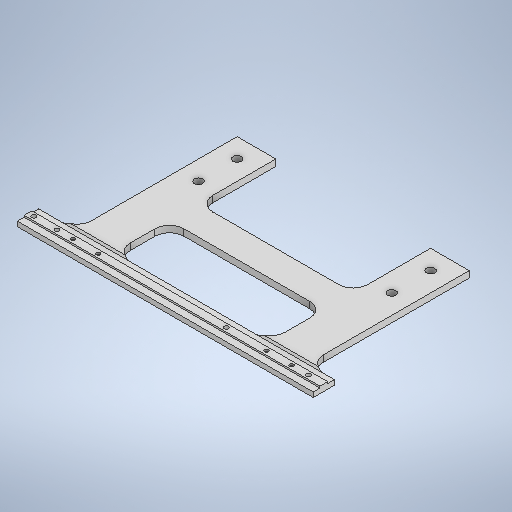
# Autodesk Inventor part: ER_Halterung_Verschraubeinheit
Saved by Autodesk Inventor 2025.2 (Build 292293000, 293)
## iProperties
Created: 2025-06-21
Part Number: ER_Halterung_Verschraubeinheit
Material: Generic
Document SubType Name: Modeling
Designer: Erik
Density: 1 g/cm^3
Appearance: Default
Author: Erik
Autodesk Inventor part; units mm, degrees
ref_plane "YZ Plane" through (0, 0, 0) normal (1, 0, 0) x (0, 1, 0)
ref_plane "XZ Plane" through (0, 0, 0) normal (0, 1, 0) x (-1, 0, 0)
ref_plane "XY Plane" through (0, 0, 0) normal (0, 0, 1) x (1, 0, 0)
sketch "Sketch1" plane through (0, 0, 0) normal (0, 1, 0) x (-1, 0, 0)
  line L0 (-153, 11) -> (153, 11)
  line L1 (153, 11) -> (153, -11)
  line L2 (153, -11) -> (-153, -11)
  line L3 (-153, -11) -> (-153, 11)
  line L4 (-153, 11) -> (153, -11) construction
  line L5 (153, 11) -> (-153, -11) construction
  point P0 (0, 0)
  dimension "d0" = 306
  dimension "d1" = 22
  constraints: 12 end point, 2 midpoint, 2 parallel, 1 horizontal, 1 perpendicular
  measures "d0" distance of L0.start L0.end
  measures "d1" distance of L0.end L1.end
extrude "Extrusion1" add sketch "Sketch1" along normal blind 5
sketch "Sketch2" plane through (0, 5, 0) normal (0, 1, 0) x (1, 0, 0)
  line L0 (-153, 11) -> (-153, -11) projected
  line L1 (153, -4) -> (-153, -4)
  line L2 (-153, -4) -> (-153, 4)
  line L3 (-153, 4) -> (153, 4)
  line L4 (153, 4) -> (153, -4)
  line L5 (153, -4) -> (-153, 4) construction
  line L6 (-153, -4) -> (153, 4) construction
  point P0 (0, 0)
  point P1 (-153, -4)
  dimension "d4" = 8
  constraints: 12 end point, 2 midpoint, 2 parallel, 1 horizontal, 1 perpendicular, 1 point on line
  measures "d4" distance between parallel lines of L3 L1
extrude "Extrusion2" add sketch "Sketch2" along normal blind 1.7
sketch "Sketch3" plane through (0, 0, 0) normal (0, -1, 0) x (1, 0, 0)
  line L0 (153, -11) -> (-153, -11) projected
  line L1 (-113, -11) -> (-73, -11)
  line L2 (-73, -11) -> (-73, -71)
  line L3 (-73, -71) -> (-113, -71)
  line L4 (-113, -71) -> (-113, -11)
  line L5 (-153, -11) -> (-153, 11) projected
  line L6 (0, 27.4) -> (0, -87.4) projected
  line L7 (113, -11) -> (73, -11)
  line L8 (153, -11) -> (153, 11)
  line L9 (113, -11) -> (73, -11)
  line L10 (73, -11) -> (73, -71)
  line L11 (73, -71) -> (113, -71)
  line L12 (113, -71) -> (113, -11)
  point P0 (0, 0)
  point P1 (-73, -11)
  point P2 (153, 0)
  dimension "d7" = 40
  dimension "d8" = 60
  dimension "d9" = 40
  dimension "d23" = 40
  dimension "d24" = 60
  dimension "d25" = 40
  constraints: 20 end point, 4 parallel, 3 symmetric about line, 2 horizontal, 2 perpendicular, 2 point on line, 1 midpoint
  measures "d7" distance of L2.end L3.end
  measures "d8" distance of L1.end L2.end
  measures "d9" distance between parallel lines of L5 L4
  measures "d23" distance of L11.end L10.end
  measures "d24" distance of L10.end L9.end
  measures "d25" distance from line of point (153, 0) L12
extrude "Extrusion3" [suppressed]
sketch "Sketch4" plane through (0, 0, 0) normal (0, -1, 0) x (1, 0, 0)
  line L0 (-153, -11) -> (-153, 11) projected
  point P0 (0, 0)
  point P1 (-147, 0)
  point P2 (-123, 0)
  point P3 (52, 0)
  point P4 (137, 0)
  dimension "d12" = 6
  dimension "d13" = 24
  dimension "d14" = 175
  dimension "d15" = 85
  measures "d12" distance from line of L0 point (-147, 0)
  measures "d13" distance of point (-123, 0) point (-147, 0)
  measures "d14" distance of point (52, 0) point (-123, 0)
  measures "d15" distance of point (137, 0) point (52, 0)
hole "Hole1" at (-147, 0, 0) at (-123, 0, 0) at (52, 0, 0) at (137, 0, 0) direction (0, 1, 0) diameter 4.5 end through all
sketch "Sketch5" plane through (0, 0, 0) normal (0, -1, 0) x (1, 0, 0)
  line L0 (153, 11) -> (153, -11) projected
  line L1 (-153, -11) -> (-153, 11) projected
  point P0 (0, 0)
  point P1 (-80.3, 0)
  point P2 (-106.3, 0)
  point P3 (-153, 0)
  dimension "d27" = 26
  dimension "d38" = 46.7
  constraints: 1 midpoint
  measures "d27" distance of point (-80.3, 0) point (-106.3, 0)
  measures "d38" distance of point (-153, 0) point (-106.3, 0)
hole "Hole2" at (-80.3, 0, 0) at (-106.3, 0, 0) direction (0, 1, 0) diameter 4.134 depth 6.7 thread size "M5x0.8" class "6H" standard "ISO Metric profile"
pattern_linear "Rectangular Pattern1" count 2 spacing 200 along (1, 0, 0) of "Hole2"
sketch "Sketch6" plane through (0, 0, 0) normal (0, -1, 0) x (1, 0, 0)
  line L0 (-113.3, 11) -> (-73.3, 11)
  line L1 (-73.3, 11) -> (-73.3, -176.642)
  line L2 (-73.3, -176.642) -> (-113.3, -176.642)
  line L3 (-113.3, -176.642) -> (-113.3, 11)
  circle A0 centre (-123, 0) radius 2.25 projected
  line L4 (-153, 11) -> (153, 11) projected
  line L5 (86.7, 11) -> (126.7, 11)
  line L6 (126.7, 11) -> (126.7, -176.642)
  line L7 (126.7, -176.642) -> (86.7, -176.642)
  line L8 (86.7, -176.642) -> (86.7, 11)
  circle A1 centre (119.7, 0) radius 2.067 projected
  circle A2 centre (-106.3, 0) radius 2.067 projected
  point P0 (0, 0)
  dimension "d39" = 40
  dimension "d41" = 187.642
  dimension "d42" = 40
  dimension "d44" = 7
  dimension "d47" = 7
  constraints: 16 end point, 4 parallel, 3 collinear, 2 horizontal, 2 perpendicular, 1 point on line
  measures "d39" distance of L1.end L2.end
  measures "d41" distance between parallel lines of L0 L2
  measures "d42" distance of L6.end L7.end
  measures "d44" distance from line of A1.centre L6
  measures "d47" horizontal distance of L0.start A2.centre
extrude "Extrusion4" add sketch "Sketch6" against normal up to surface (5 mm away) contours L0 L1 L2 L3 | L4 L6 L7 L8 | A1 | A2
sketch "Sketch7" plane through (0, 0, 0) normal (0, -1, 0) x (1, 0, 0)
  line L0 (-73.3, -176.642) -> (-73.3, -11) projected
  line L1 (-113.3, -176.642) -> (-73.3, -176.642) projected
  point P0 (0, 0)
  point P1 (-93.3, -156.642)
  point P2 (-93.3, -116.642)
  dimension "d48" = 20
  dimension "d49" = 20
  dimension "d50" = 20
  dimension "d51" = 40
  measures "d48" distance from line of L0 point (-93.3, -156.642)
  measures "d49" distance from line of L0 point (-93.3, -116.642)
  measures "d50" distance from line of L1 point (-93.3, -156.642)
  measures "d51" distance of point (-93.3, -156.642) point (-93.3, -116.642)
hole "Hole3" at (-93.3, 0, -156.642) at (-93.3, 0, -116.642) direction (0, 1, 0) diameter 8.6 end through all
pattern_linear "Rectangular Pattern2" count 2 spacing 200 along (1, 0, 0) of "Hole3"
sketch "Skizze8" plane through (0, 5, 0) normal (0, 1, 0) x (1, 0, 0)
  circle A0 centre (106.7, 116.642) radius 4.3 projected
  circle A1 centre (106.7, 156.642) radius 4.3 projected
  circle A2 centre (-93.3, 116.642) radius 4.3 projected
  circle A3 centre (-93.3, 156.642) radius 4.3 projected
  line L0 (-153, 4) -> (153, 4) projected
  line L1 (153, 4) -> (153, 11) projected
  line L2 (153, 11) -> (126.7, 11) projected
  line L3 (126.7, 176.642) -> (126.7, 11) projected
  line L4 (86.7, 176.642) -> (126.7, 176.642) projected
  line L5 (86.7, 11) -> (86.7, 176.642) projected
  line L6 (86.7, 11) -> (-73.3, 11) projected
  line L7 (-73.3, 176.642) -> (-73.3, 11) projected
  line L8 (-113.3, 176.642) -> (-73.3, 176.642) projected
  line L9 (-113.3, 11) -> (-113.3, 176.642) projected
  line L10 (-113.3, 11) -> (-153, 11) projected
  line L11 (-153, 11) -> (-153, 4) projected
  line L12 (-113.3, 11) -> (126.7, 11)
  line L13 (126.7, 11) -> (126.7, 176.642)
  line L14 (126.7, 176.642) -> (-113.3, 176.642)
  line L15 (-113.3, 176.642) -> (-113.3, 11)
  point P0 (0, 0)
  point P1 (126.7, 11)
  constraints: 8 end point, 2 parallel, 1 horizontal, 1 perpendicular
extrude "Extrusion5" add sketch "Skizze8" along normal up to surface (1.7 mm away) contours L9 L8 L7 L12 | L12 L5 L4 L3
chamfer "Fasen1" distance 1.7 angle 45 2 edges at (-93.3, 6.7, -11) (106.7, 6.7, -11)
sketch "Skizze9" plane through (-73.3, 0, -11) normal (1, 0, 0) x (0, 0, -1)
  line L0 (1.7, 6.7) -> (165.642, 6.7) projected
  line L1 (0, 0) -> (165.642, 0) projected
  line L2 (55.642, 6.7) -> (85.642, 6.7)
  line L3 (85.642, 6.7) -> (85.642, 0)
  line L4 (85.642, 0) -> (55.642, 0)
  line L5 (55.642, 0) -> (55.642, 6.7)
  line L6 (165.642, 0) -> (165.642, 6.7) projected
  point P0 (-11, 0)
  dimension "d67" = 80
  dimension "d68" = 30
  constraints: 8 end point, 2 parallel, 2 point on line, 1 horizontal, 1 perpendicular
  measures "d67" distance between parallel lines of L3 L6
  measures "d68" distance between parallel lines of L3 L5
extrude "Extrusion6" add sketch "Skizze9" along normal up to surface (160 mm away) contours L0 L3 L1 L5
fillet "Rundung1" radius 15 12 edges at (-73.3, 3.35, -66.642) (86.7, 3.35, -66.642) (86.7, 3.35, -96.642) (-73.3, 3.35, -96.642) (-113.3, 5, -11) (-113.3, 2.5, -11) (-73.3, 2.5, -11) (-73.3, 5, -11) (126.7, 5, -11) (126.7, 2.5, -11) (86.7, 5, -11) (86.7, 2.5, -11)
equation "\"d44\" = d40"
equation "\"d40\" = 7"
body "Solid1"
